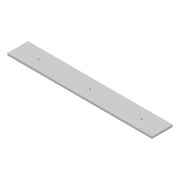
# Autodesk Inventor part: Lid_SidePanel
Saved by Autodesk Inventor 2016 (Build 200138000, 138)
## iProperties
Created: 2014-11-24
Part Number: Lid_SidePanel
Material: Polycarbonat, klar
Document SubType Name: Modeling
Designer: Gero Hofmann
Density: 1.2 g/cm^3
Appearance: Polycarbonat - klar
Author: Gero Hofmann
Autodesk Inventor part; units mm, degrees
ref_plane "YZ Plane" through (0, 0, 0) normal (1, 0, 0) x (0, 1, 0)
ref_plane "XZ Plane" through (0, 0, 0) normal (0, 1, 0) x (-1, 0, 0)
ref_plane "XY Plane" through (0, 0, 0) normal (0, 0, 1) x (1, 0, 0)
sketch "Skizze1" plane through (0, 0, 0) normal (0, 0, 1) x (1, 0, 0)
  line L0 (0, 0) -> (700, 0)
  line L1 (700, 0) -> (700, 100)
  line L2 (700, 100) -> (0, 100)
  line L3 (0, 100) -> (0, 0)
  dimension "d4" = 700
  dimension "d5" = 100
  constraints: 8 end point, 2 parallel, 1 horizontal, 1 perpendicular
  measures "d4" distance of L0.start L0.end
  measures "d5" distance of L2.end L0.start
extrude "Extrusion1" add sketch "Skizze1" along normal blind 10
sketch "Skizze2" plane through (0, 0, 0) normal (0, 0, -1) x (-1, 0, 0)
  line L0 (736.2089, -6.1125) -> (736.2089, 106.1125)
  line L1 (-100, 50) -> (-600, 50) construction
  line L2 (0, 0) -> (-700, 0) projected
  line L3 (0, 100) -> (0, 0) projected
  point P0 (-350, 50)
  point P1 (736.2089, 50)
  point P2 (-350, 0)
  point P3 (-350, 0)
  point P4 (-350, 0)
  point P5 (0, 50)
  dimension "d6" = 500
  constraints: 6 midpoint, 4 end point, 2 horizontal alignment, 1 coincident, 1 horizontal, 1 vertical alignment
  measures "d6" distance of L1.start L1.end
hole "Bohrung1" at (100, 50, 0) at (350, 50, 0) at (600, 50, 0) direction (0, 0, 1) diameter 6.6 end through all countersink diameter 14.5 countersink angle 90 clearance for "Innensechskant-Senkkopfschraube DIN EN ISO 10642" size "M6" standard "DIN"
